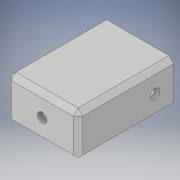
# Autodesk Inventor part: Pernotta
Saved by Autodesk Inventor 2019.1 (Build 231200000, 200)
## iProperties
Created: 2019-08-01
Part Number: Pernotta
Material: Genérico
Document SubType Name: Modeling
Designer: IEEE UFABC
Density: 1 g/cm^3
Appearance: Padrão
Author: IEEE UFABC
Autodesk Inventor part; units mm, degrees
ref_plane "YZ Plane" through (0, 0, 0) normal (1, 0, 0) x (0, 1, 0)
ref_plane "XZ Plane" through (0, 0, 0) normal (0, 1, 0) x (-1, 0, 0)
ref_plane "XY Plane" through (0, 0, 0) normal (0, 0, 1) x (1, 0, 0)
sketch "Esboço1" plane through (0, 0, 0) normal (0, 1, 0) x (-1, 0, 0)
  line L0 (9.4987, -2.4377) -> (-20.5013, -2.4377)
  line L1 (-20.5013, -2.4377) -> (-20.5013, -42.4377)
  line L2 (-20.5013, -42.4377) -> (9.4987, -42.4377)
  line L3 (9.4987, -42.4377) -> (9.4987, -2.4377)
  point P0 (0, 0)
  dimension "d0" = 30
  dimension "d1" = 40
  constraints: 8 end point, 2 parallel, 1 horizontal, 1 perpendicular
  measures "d0" distance of L2.end L1.end
  measures "d1" distance of L1.end L0.end
extrude "Extrusão1" add sketch "Esboço1" along normal blind 18
sketch "Esboço2" plane through (20.5013, 0, -42.4377) normal (0, 0, -1) x (-1, 0, 0)
  line L0 (28, 2) -> (2, 2)
  line L1 (2, 2) -> (2, 16)
  line L2 (2, 16) -> (28, 16)
  line L3 (28, 16) -> (28, 2)
  line L4 (0, 0) -> (30, 0) projected
  line L5 (0, 18) -> (30, 18) projected
  line L6 (0, 0) -> (0, 18) projected
  line L7 (30, 0) -> (30, 18) projected
  point P0 (20.5013, 0)
  dimension "d4" = 2
  dimension "d5" = 2
  dimension "d6" = 2
  dimension "d7" = 2
  constraints: 8 end point, 2 parallel, 1 horizontal, 1 perpendicular
  measures "d4" distance between parallel lines of L0 L4
  measures "d5" distance between parallel lines of L5 L2
  measures "d6" distance between parallel lines of L6 L1
  measures "d7" distance between parallel lines of L7 L3
extrude "Extrusão2" cut sketch "Esboço2" against normal blind 38 contours L0 L1 L2 L3
chamfer "Chanfro1" distance 2 angle 45 7 edges at (-9.4987, 18, -22.4377) (-9.4987, 0, -22.4377) (5.5013, 18, -2.4377) (-9.4987, 9, -2.4377) (20.5013, 18, -22.4377) (20.5013, 9, -2.4377) (20.5013, 0, -22.4377)
chamfer "Chanfro2" distance 2 angle 45 1 edges at (5.5013, 0, -2.4377)
sketch "Esboço3" plane through (0, 0, 0) normal (0, -1, 0) x (1, 0, 0)
  line L0 (-3.4987, -6.1642) -> (14.5013, -6.1642)
  line L1 (14.5013, -6.1642) -> (14.5013, -24.1642)
  line L2 (14.5013, -24.1642) -> (-3.4987, -24.1642)
  line L3 (-3.4987, -24.1642) -> (-3.4987, -6.1642)
  line L4 (-7.4987, -42.4377) -> (-7.4987, -4.4377) projected
  point P0 (0, 0)
  dimension "d16" = 18
  dimension "d17" = 18
  dimension "d18" = 4
  constraints: 8 end point, 2 parallel, 1 horizontal, 1 perpendicular
  measures "d16" distance of L1.end L2.end
  measures "d17" distance of L0.end L1.end
  measures "d18" distance between parallel lines of L4 L3
extrude "Extrusão3" cut sketch "Esboço3" against normal blind 5
sketch "Esboço4" plane through (-9.4987, 2, -42.4377) normal (-1, 0, 0) x (0, 0, 1)
  line L0 (0, 14) -> (38, 14) projected
  line L1 (7.7786, 13) -> (0, 13)
  line L2 (7.7786, 1) -> (0, 1)
  line L3 (0, 0) -> (0, 14) projected
  ellipse E0 centre (13.7786, 7) end of major axis (13.7786, 10) minor radius 3.3 (13.0203, 4.0803) -> (13.0203, 9.9197) ccw
  arc A0 (7.7786, 1) -> (13.0203, 4.0803) centre (7.7786, 7) ccw
  arc A1 (13.0203, 9.9197) -> (7.7786, 13) centre (7.7786, 7) ccw
  circle A2 centre (7.7786, 7) radius 2
  point P0 (42.4377, -2)
  dimension "d23" = 3.3
  dimension "d24" = 3
  dimension "d22" = 7
  dimension "d25" = 4
  constraints: 4 end point, 4 point on circle, 3 centre point, 2 horizontal, 1 coincident, 1 point on line, 4 other
  measures "d22" distance from line of L0 A0.centre
  measures "d25" diameter of A2
extrude "Extrusão4" cut sketch "Esboço4" against normal blind 5
sketch "Esboço5" plane through (-9.4987, 9, -34.6591) normal (-1, 0, 0) x (0, 0, 1)
  circle A0 centre (0, 0) radius 2 projected
  circle A1 centre (0, 0) radius 2
  point P0 (34.6591, -9)
  constraints: 1 centre point, 1 coincident
extrude "Extrusão5" cut sketch "Esboço5" against normal blind 69
sketch "Esboço6" plane through (-7.4987, 16, -2.4377) normal (0, 0, 1) x (1, 0, 0)
  line L0 (0, -4) -> (0, -10) construction
  line L1 (0, -7) -> (26, -7) construction
  line L2 (26, -9) -> (26, -5) construction
  line L3 (22, -14) -> (4, -14) construction
  line L4 (13, -14) -> (13, 0) construction
  line L5 (26, 0) -> (0, 0) construction
  circle A0 centre (13, -7) radius 2
  point P0 (7.4987, -16)
  point P1 (0, -9.9197)
  point P2 (0, -4.0803)
  dimension "d30" = 4
  constraints: 5 midpoint, 4 end point, 1 centre point
  measures "d30" diameter of A0
extrude "Extrusão6" cut sketch "Esboço6" against normal blind 10
